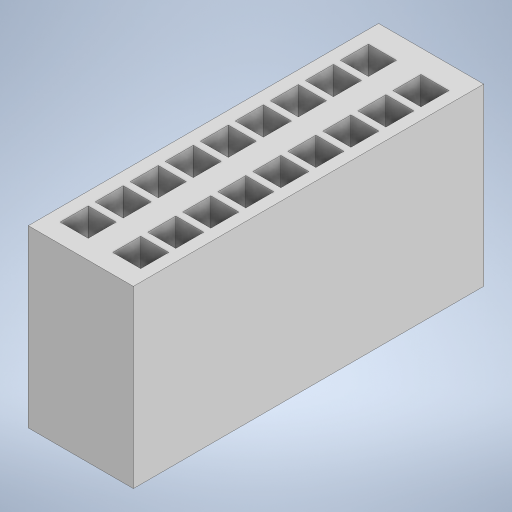
# Autodesk Inventor part: 矩形陣列
Saved by Autodesk Inventor 2024.2 (Build 282272000, 272)
## iProperties
Created: 2024-05-02
Part Number: 矩形陣列
Material: 一般
Document SubType Name: Modeling
Designer: User
Density: 1 g/cm^3
Appearance: 預設
Author: User
Autodesk Inventor part; units mm, degrees
ref_plane "YZ Plane" through (0, 0, 0) normal (1, 0, 0) x (0, 1, 0)
ref_plane "XZ Plane" through (0, 0, 0) normal (0, 1, 0) x (-1, 0, 0)
ref_plane "XY Plane" through (0, 0, 0) normal (0, 0, 1) x (1, 0, 0)
sketch "草圖1" plane through (0, 0, 0) normal (0, 1, 0) x (-1, 0, 0)
  line L0 (0, 0) -> (30, 0)
  line L1 (30, 0) -> (30, -100)
  line L2 (30, -100) -> (0, -100)
  line L3 (0, -100) -> (0, 0)
  dimension "d0" = 30
  dimension "d1" = 100
  constraints: 8 end point, 2 parallel, 1 horizontal, 1 perpendicular
  measures "d0" distance of L1.end L2.end
  measures "d1" distance of L0.end L1.end
extrude "擠出1" add sketch "草圖1" along normal blind 50
sketch "草圖2" plane through (0, 50, 0) normal (0, 1, 0) x (1, 0, 0)
  line L0 (-11.3304, 13.4262) -> (-3.3304, 13.4262)
  line L1 (-3.3304, 13.4262) -> (-3.3304, 5.4262)
  line L2 (-3.3304, 5.4262) -> (-11.3304, 5.4262)
  line L3 (-11.3304, 5.4262) -> (-11.3304, 13.4262)
  point P0 (0, 0)
  dimension "d4" = 8
  dimension "d5" = 8
  constraints: 8 end point, 2 parallel, 1 horizontal, 1 perpendicular
  measures "d4" distance of L1.end L2.end
  measures "d5" distance of L0.end L1.end
extrude "擠出2" cut sketch "草圖2" against normal blind 50
pattern_linear "矩形陣列1" count 9 spacing 10 along (0, 0, -1) of "擠出2"
pattern_linear "矩形陣列2" count 2 spacing 15 along (-1, 0, 0) of "擠出2", "矩形陣列1"
